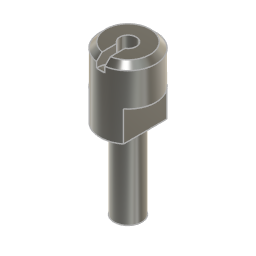
_thread_guide.b8f5327d-0b44-4c44-950b-1926ca93f7ff (Autodesk Fusion 360 design; units mm, degrees)
Autodesk Fusion 360 part; units mm, degrees
sketch "Sketch1" plane through (0, 0, 0) normal (0, 0, 1) x (1, 0, 0)
  circle A0 centre (0, 0) radius 2.5
  circle A1 centre (0, 0) radius 1.5
  dimension "d1" = 5
  dimension "d2" = 3
  constraint coincident A0.centre A1.centre
  measures "d1" diameter of A0
  measures "d2" diameter of A1
extrude "Extrude1" add sketch "Sketch1" along normal blind 20
sketch "Sketch2" plane through (0, 0, 20) normal (0, 0, 1) x (-1, 0, 0)
  circle A0 centre (0, 0) radius 1.5
  circle A1 centre (0, 0) radius 2.5
  circle A2 centre (0, 0) radius 5
  dimension "d5" = 2.5
  constraint coincident A0.centre A1.centre
  measures "d5" distance of A1 A2
extrude "Extrude2" add sketch "Sketch2" along normal blind 7 contours A1 | A2
sketch "Sketch3" plane through (0, 0, 0) normal (0, 1, 0) x (1, 0, 0)
  line L0 (-5, -27) -> (5, -27)
  line L1 (0, -27) -> (0, -20) construction
  line L2 (-5, -20) -> (5, -20)
  line L3 (-0.75, -27) -> (0.75, -27)
  line L4 (0.75, -27) -> (0.75, -25)
  line L5 (0.75, -25) -> (-0.75, -25)
  line L6 (-0.75, -25) -> (-0.75, -27)
  dimension "d8" = 1.5
  dimension "d9" = 2
  constraint midpoint L0 L1.start
  constraint perpendicular L0 L1
  constraint midpoint L1.end L2
  constraint horizontal L3
  constraint vertical L4
  constraint horizontal L5
  constraint vertical L6
  constraint coincident L0 L3.start
  constraint symmetric L1 L4.end L5.end
  measures "d8" distance of L4.end L5.end
  measures "d9" distance of L3.start L5.end
extrude "Extrude3" cut sketch "Sketch3" against normal blind 6
sketch "Sketch4" plane through (0, 0, 0) normal (1, 0, 0) x (0, 1, 0)
  line L0 (-1.299, 27) -> (-4.9434, 27)
  line L1 (-1.299, 27) -> (1.5, 27)
  line L2 (-1.299, 25) -> (-4.9434, 25)
  line L3 (-1.299, 25) -> (-1.299, 23.4446)
  arc A0 (-1.299, 23.4446) -> (-4.9434, 25) centre (-4.9434, 19.9527) ccw
  constraint coincident L2.start L3.start
  constraint perpendicular L2 L3
  constraint tangent L2 A0
  constraint coincident L2.end A0.end
extrude "Extrude4" cut sketch "Sketch4" along normal blind 0.75 and the other way blind 0.75
chamfer "Chamfer1" distance 1 angle 45 1 edges at (0, 5, 27)
sketch "Sketch5" plane through (0, 0, 20) normal (0, 0, -1) x (1, 0, 0)
  circle A0 centre (0, 0) radius 5
  circle A1 centre (0, 0) radius 2.5
  circle A2 centre (0, 0) radius 5
  line L0 (-3.1, 3.923) -> (-3.1, -3.923)
  line L1 (3.1, 3.923) -> (3.1, -3.923)
  line L2 (0, -5) -> (0, 5) construction
  dimension "d19" = 6.2
  constraint coincident A2 L0.start
  constraint coincident A2 L0.end
  constraint vertical L0
  constraint coincident A2 L1.start
  constraint coincident A2 L1.end
  constraint parallel L0 L1
  constraint coincident A2 L2.start
  constraint coincident A2 L2.end
  constraint vertical L2
  constraint coincident A0.centre L2
  measures "d19" distance of L0 L1
extrude "Extrude5" add sketch "Sketch5" along normal blind 5.5 contours A0 A2 L0 L1
